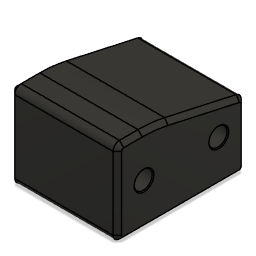
bumper block v1 (Autodesk Fusion 360 design; units mm, degrees)
Autodesk Fusion 360 part; units mm, degrees
sketch "Sketch1" plane through (0, 0, 0) normal (1, 0, 0) x (0, 0, -1)
  line L0 (0, 0) -> (0, 40)
  line L1 (0, 40) -> (18, 40)
  line L2 (18, 40) -> (60, 30.6888)
  line L3 (0, 0) -> (60, 0)
  line L4 (60, 0) -> (60, 30.6888)
  dimension "d1" = 40
  dimension "d2" = 18
  dimension "d3" = 12.5
  dimension "d4" = 60
  constraint coincident L0.start L3.start
  constraint vertical L0
  constraint perpendicular L0 L1
  constraint perpendicular L0 L3
  constraint vertical L4
  measures "d1" distance of L0.start L0.end
  measures "d2" distance of L0.end L1.end
  measures "d3" angle of L2 L3
  measures "d4" distance of L0.start L3.end
extrude "Extrude1" add sketch "Sketch1" along normal blind 50 makes body 1
sketch "Sketch2" plane through (0, 0, 0) normal (-1, 0, 0) x (0, 0, 1)
  line L0 (-60, 0) -> (0, 0)
  line L1 (0, 0) -> (0, 40)
  line L2 (0, 40) -> (-18, 40)
  line L3 (-18, 40) -> (-60, 30.6888)
  line L4 (-60, 30.6888) -> (-60, 0)
  circle A0 centre (-47.5, 20) radius 4.25
  line L5 (-60, 20) -> (0, 20) construction
  circle A1 centre (-12.5, 20) radius 4.25
  circle A2 centre (-47.5, 20) radius 7.25
  circle A3 centre (-12.5, 20) radius 7.25
  dimension "d9" = 8.5
  dimension "d12" = 12.5
  dimension "d13" = 12.5
  dimension "d14" = 14.5
  dimension "d15" = 20
  constraint coincident L4 L5.start
  constraint coincident L1 L5.end
  constraint perpendicular L1 L5
  constraint coincident A0.centre L5
  constraint coincident L5 A1.centre
  constraint equal A0 A1
  constraint concentric A0 A2
  constraint concentric A1 A3
  constraint equal A2 A3
  measures "d9" diameter of A0
  measures "d12" distance of L1 A1.centre
  measures "d13" distance of L4 A0.centre
  measures "d14" diameter of A2
  measures "d15" distance of L0 L5
extrude "Extrude2" cut sketch "Sketch2" against normal blind 63 contours A0 | A1 bodies 1
fillet "Fillet1" radius 57.5 1 edges at (25, 40, -18) on bodies 1
fillet "Fillet1" radius 3 4 edges at (25, 30.6888, -60) (25, 40, 0) (25, 0, 0) (25, 0, -60) on bodies 1
chamfer "Chamfer1" distance 0.4 angle 45 2 faces at (16.6667, 19.5768, -8.2711) (16.6667, 19.5768, -43.2711) on bodies 1
chamfer "Chamfer1" distance 2 angle 45 10 faces at (16.6667, 36.1613, -35.3151) (16.6667, 28.9517, -59.9241) (33.3333, 11.427, -60) (16.6667, 1.1455, -59.3582) (33.3333, 0, -21) (16.6667, 0.0034, -2.8573) (16.6667, 14.3333, 0) (16.6667, 38.3747, -0.3335) (16.6667, 40, -5.9009) (16.6667, 39.5782, -18.6549) on bodies 1
copy_body "Body->Comp1" bodies 1 removing the originals makes body 2 in component "bumper block"
component "bumper block" placed x (1, 0, 0) y (0, 1, 0) z (0, 0, 1) at (0, 0, 0)
named bodies: "bumper block"
